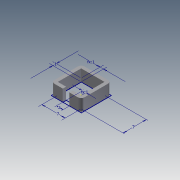
# Autodesk Inventor part: cable_clip_rev1
Saved by Autodesk Inventor 2011 (Build 150239000, 239)
## iProperties
Created: 2013-02-14
Part Number: cable_clip_rev1
Document SubType Name: Modeling
Designer: Administrator
Density: 1 g/cm^3
Author: Administrator
Autodesk Inventor part; units mm, degrees
ref_plane "YZ Plane" through (0, 0, 0) normal (1, 0, 0) x (0, 1, 0)
ref_plane "XZ Plane" through (0, 0, 0) normal (0, 1, 0) x (-1, 0, 0)
ref_plane "XY Plane" through (0, 0, 0) normal (0, 0, 1) x (1, 0, 0)
sketch "Sketch1" plane through (0, 0, 0) normal (0, 0, 1) x (1, 0, 0)
  line L0 (-3.5, 3.5) -> (3.5, 3.5)
  line L1 (3.5, 3.5) -> (3.5, -3.5)
  line L2 (3.5, -3.5) -> (-3.5, -3.5)
  line L3 (-3.5, -3.5) -> (-3.5, 3.5)
  line L4 (-4.5, 4.5) -> (4.5, 4.5)
  line L5 (4.5, 4.5) -> (4.5, -4.5)
  line L6 (4.5, -4.5) -> (-4.5, -4.5)
  line L7 (-4.5, -4.5) -> (-4.5, 4.5)
  line L8 (-1, -3.5) -> (-1, -4.5)
  line L9 (1, -3.5) -> (1, -4.5)
  point P0 (0, 0)
  point P1 (0, 3.5)
  point P2 (-3.5, 0)
  point P3 (-4.5, 0)
  point P4 (0, 4.5)
  dimension "d0" = 1
  dimension "d1" = 1
  dimension "d2" = 7
  dimension "d3" = 7
  dimension "d4" = 2
  dimension "d5" = 1
  constraints: 20 end point, 4 midpoint, 4 parallel, 4 perpendicular, 4 point on line, 2 horizontal, 2 horizontal alignment, 2 vertical alignment
  measures "d0" distance between parallel lines of L4 L0
  measures "d1" distance between parallel lines of L7 L3
  measures "d2" distance between parallel lines of L1 L3
  measures "d3" distance between parallel lines of L2 L0
  measures "d4" distance between parallel lines of L9 L8
  measures "d5" distance from line of point (0, 0) L8
extrude "Extrusion1" add sketch "Sketch1" along normal blind 3.5 contours L3 L2 L8 L6 L7 L4 L5 L9 L1 L0
fillet "Fillet1" radius 1 4 edges at (4.5, 4.5, 1.75) (-4.5, 4.5, 1.75) (-4.5, -4.5, 1.75) (4.5, -4.5, 1.75)
equation "\"d1\" = d0"
equation "\"d5\" = 0.5 * d4"
body "Solid1"
